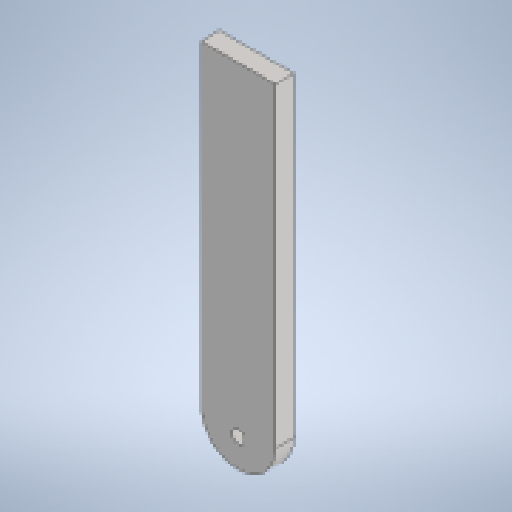
# Autodesk Inventor part: шатун2
Saved by Autodesk Inventor 2023.1 (Build 271208000, 208)
## iProperties
Created: 2024-12-17
Part Number: шатун2
Material: Типовые
Document SubType Name: Modeling
Designer: DELL
Density: 1 g/cm^3
Appearance: По умолчанию
Author: DELL
Autodesk Inventor part; units mm, degrees
ref_plane "YZ Plane" through (0, 0, 0) normal (1, 0, 0) x (0, 1, 0)
ref_plane "XZ Plane" through (0, 0, 0) normal (0, 1, 0) x (-1, 0, 0)
ref_plane "XY Plane" through (0, 0, 0) normal (0, 0, 1) x (1, 0, 0)
sketch "Эскиз1" plane through (0, 0, 0) normal (0, 0, 1) x (1, 0, 0)
  circle A0 centre (0, 0) radius 9 projected
  circle A1 centre (0, 0) radius 5 projected
  circle A2 centre (0, 0) radius 1.65 projected
  point P0 (0, 0)
extrude "Выдавливание1" add sketch "Эскиз1" along normal blind 3.2363 contours A0
sketch "Эскиз2" plane through (0, 0, 3.2363) normal (0, 0, 1) x (1, 0, 0)
  line L0 (0, -7.7644) -> (0, 107) construction
  line L1 (10, 2.2356) -> (10, 97)
  line L2 (-10, 97) -> (-10, 2.2356)
  arc A0 (-10, 2.2356) -> (10, 2.2356) centre (0, 2.2356) ccw
  arc A1 (10, 97) -> (-10, 97) centre (0, 97) ccw
  line L3 (343.1024, 87) -> (-136.8976, 87) projected
  circle A2 centre (0, 0) radius 5 construction
  circle A3 centre (0, 0) radius 1.65
  point P0 (0, 0)
  point P1 (0, 49.6178)
  point P2 (0, 107)
  point P3 (10, 87)
  point P4 (-10, 87)
  dimension "d2" = 20
  dimension "d3" = 20
  dimension "d4" = 3.3
  constraints: 8 end point, 7 point on circle, 4 tangent, 3 centre point, 2 point on line, 1 coincident, 1 midpoint, 1 parallel, 1 vertical
  measures "d2" diameter of A1
  measures "d3" distance from line of L3 point (0, 107)
  measures "d4" diameter of A3
extrude "Выдавливание2" add sketch "Эскиз2" along normal blind 5 contours A0 L2 L3 L1
